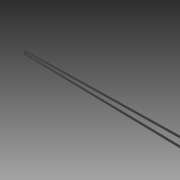
# Autodesk Inventor part: x_axis_belt
Saved by Autodesk Inventor 2014 (Build 180170000, 170)
## iProperties
Created: 2014-03-26
Part Number: x_axis_belt
Material: Rubber
Document SubType Name: Modeling
Designer: buben
Density: 0.93 g/cm^3
Appearance: Rubber - Black - Version 1.1
Author: buben
Autodesk Inventor part; units mm, degrees
ref_plane "YZ Plane" through (0, 0, 0) normal (1, 0, 0) x (0, 1, 0)
ref_plane "XZ Plane" through (0, 0, 0) normal (0, 1, 0) x (-1, 0, 0)
ref_plane "XY Plane" through (0, 0, 0) normal (0, 0, 1) x (1, 0, 0)
sketch "Sketch1" plane through (0, 0, 0) normal (0, 1, 0) x (-1, 0, 0)
  line L0 (0.0672, -6.0996) -> (-626.6479, -12.9992)
  line L1 (0.0672, 6.0996) -> (-626.6479, 12.9992)
  arc A0 (0.0672, -6.0996) -> (0.0672, 6.0996) centre (0, 0) ccw
  arc A1 (-626.6479, 12.9992) -> (-626.6479, -12.9992) centre (-626.791, 0) ccw
  line L2 (-626.6327, 14.3791) -> (0.0823, 7.4795)
  arc A2 (0.0823, -7.4795) -> (0.0823, 7.4795) centre (0, 0) ccw
  line L3 (0.0823, -7.4795) -> (-626.6327, -14.3791)
  arc A3 (-626.6327, 14.3791) -> (-626.6327, -14.3791) centre (-626.791, 0) ccw
  dimension "d2" = 6.1
  dimension "d3" = 13
  dimension "d4" = 1.38
  dimension "d5" = 626.791
  constraints: 8 end point, 8 point on circle, 4 centre point, 4 tangent, 1 coincident, 1 horizontal alignment, 3 other
  measures "d2" radius of A0
  measures "d3" radius of A1
  measures "d4" distance between parallel lines of L2 L1
  measures "d5" distance of A1.centre point (0, 0)
extrude "Extrusion1" add sketch "Sketch1" along normal blind 6
chamfer "Chamfer1" distance 0.2 angle 45 16 edges at (313.2904, 6, 9.5494) (-6.1, 6, 0) (313.2904, 6, -9.5494) (639.791, 6, 0) (313.2752, 6, 10.9293) (641.171, 6, 0) (313.2752, 6, -10.9293) (-7.48, 6, 0) (313.2752, 0, 10.9293) (-7.48, 0, 0) (313.2752, 0, -10.9293) (641.171, 0, 0) (313.2904, 0, 9.5494) (639.791, 0, 0) (313.2904, 0, -9.5494) (-6.1, 0, 0)
body "Solid1"
